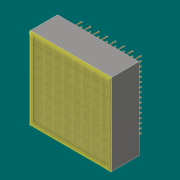
# Autodesk Inventor part: H12700A
Saved by Autodesk Inventor 2016 (Build 200138000, 138)
## iProperties
Created: 2015-10-20
Part Number: H12700A
Material: ABS Plastic
Document SubType Name: Modeling
Designer: Sawaiz
Density: 1.06 g/cm^3
Appearance: Smooth - White
Author: Sawaiz
Autodesk Inventor part; units mm, degrees
ref_plane "YZ Plane" through (0, 0, 0) normal (1, 0, 0) x (0, 1, 0)
ref_plane "XZ Plane" through (0, 0, 0) normal (0, 1, 0) x (-1, 0, 0)
ref_plane "XY Plane" through (0, 0, 0) normal (0, 0, 1) x (1, 0, 0)
sketch "Sketch1" plane through (0, 0, 0) normal (1, 0, 0) x (0, 1, 0)
  line L0 (-26, -26) -> (26, -26)
  line L1 (26, -26) -> (26, 26)
  line L2 (26, 26) -> (-26, 26)
  line L3 (-26, 26) -> (-26, -26)
  line L4 (-26, -26) -> (26, 26) construction
  line L5 (26, -26) -> (-26, 26) construction
  point P0 (0, 0)
  dimension "d0" = 52
  dimension "d1" = 52
  constraints: 12 end point, 2 midpoint, 2 parallel, 1 horizontal, 1 perpendicular
  measures "d0" distance of L2.end L1.end
  measures "d1" distance of L1.end L0.end
extrude "Extrusion1" add sketch "Sketch1" along normal blind 17.5
sketch "Sketch2" plane through (17.5, 0, 0) normal (1, 0, 0) x (0, 0, -1)
  line L0 (24.25, -24.25) -> (-24.25, -24.25)
  line L1 (-24.25, -24.25) -> (-24.25, 24.25)
  line L2 (-24.25, 24.25) -> (24.25, 24.25)
  line L3 (24.25, 24.25) -> (24.25, -24.25)
  line L4 (24.25, -24.25) -> (-24.25, 24.25) construction
  line L5 (-24.25, -24.25) -> (24.25, 24.25) construction
  point P0 (0, 0)
  dimension "d4" = 48.5
  dimension "d5" = 48.5
  constraints: 12 end point, 2 midpoint, 2 parallel, 1 horizontal, 1 perpendicular
  measures "d4" distance of L1.end L2.end
  measures "d5" distance of L0.end L1.end
extrude "Extrusion2" cut sketch "Sketch2" against normal blind 14.9
sketch "Sketch3" plane through (2.6, 0, 0) normal (1, 0, 0) x (0, 0, -1)
  line L0 (24.25, -24.25) -> (-24.25, -24.25) projected
  line L1 (24.25, 24.25) -> (24.25, -24.25) projected
  line L2 (-24.25, 24.25) -> (24.25, 24.25) projected
  line L3 (-24.25, -24.25) -> (-24.25, 24.25) projected
  line L4 (24.25, -24.25) -> (-24.25, -24.25) projected
  line L5 (-24.25, -24.25) -> (-18.1875, -24.25)
  line L6 (-18.1875, -24.25) -> (-18.1875, -18.1875)
  line L7 (-18.1875, -18.1875) -> (-24.25, -18.1875)
  line L8 (-24.25, -18.1875) -> (-24.25, -24.25)
  line L9 (-23.5764, -18.1875) -> (-22.9028, -18.1875)
  line L10 (-22.9028, -18.1875) -> (-22.9028, -24.25)
  line L11 (-22.9028, -24.25) -> (-23.5764, -24.25)
  line L12 (-23.5764, -24.25) -> (-23.5764, -18.1875)
  line L13 (-22.2292, -18.1875) -> (-21.5556, -18.1875)
  line L14 (-21.5556, -18.1875) -> (-21.5556, -24.25)
  line L15 (-21.5556, -24.25) -> (-22.2292, -24.25)
  line L16 (-22.2292, -24.25) -> (-22.2292, -18.1875)
  line L17 (-20.8819, -24.25) -> (-20.2083, -24.25)
  line L18 (-20.2083, -24.25) -> (-20.2083, -18.1875)
  line L19 (-20.2083, -18.1875) -> (-20.8819, -18.1875)
  line L20 (-20.8819, -18.1875) -> (-20.8819, -24.25)
  line L21 (-19.5347, -24.25) -> (-18.8611, -24.25)
  line L22 (-18.8611, -24.25) -> (-18.8611, -18.1875)
  line L23 (-18.8611, -18.1875) -> (-19.5347, -18.1875)
  line L24 (-19.5347, -18.1875) -> (-19.5347, -24.25)
  line L25 (-18.2875, -18.2875) -> (-18.2875, -24.15)
  line L26 (-18.2875, -24.15) -> (-24.15, -24.15)
  line L27 (-24.15, -24.15) -> (-24.15, -18.2875)
  line L28 (-24.15, -18.2875) -> (-18.2875, -18.2875)
  point P0 (0, 0)
  dimension "d8" = 6.0625
  dimension "d9" = 6.0625
  dimension "d10" = 0.6736
  dimension "d11" = 0.6736
  dimension "d12" = 0.6736
  dimension "d13" = 0.6736
  dimension "d14" = 0.6736
  dimension "d15" = 0.6736
  dimension "d16" = 0.6736
  dimension "d17" = 0.6736
  dimension "d18" = 0.1
  constraints: 48 end point, 12 parallel, 8 point on line, 6 perpendicular, 5 horizontal, 3 other
  measures "d8" distance of L7.end L6.end
  measures "d9" distance of L6.end L5.end
  measures "d10" distance between parallel lines of L8 L12
  measures "d11" distance between parallel lines of L10 L12
  measures "d12" distance between parallel lines of L10 L16
  measures "d13" distance between parallel lines of L16 L14
  measures "d14" distance between parallel lines of L14 L20
  measures "d15" distance between parallel lines of L20 L18
  measures "d16" distance between parallel lines of L18 L24
  measures "d17" distance between parallel lines of L24 L22
  measures "d18" distance between parallel lines of L6 L25
extrude "Extrusion3" add sketch "Sketch3" along normal blind 13.9 separate body contours L0 L24 L26 L22 | L26 L24 L28 L22 | L22 L28 L24 L7 | L0 L20 L26 L18 | L7 L10 L28 L12 | L26 L20 L28 L18 | L18 L28 L20 L7 | L12 L26 L10 L0 | L28 L10 L26 L12 | L0 L16 L26 L14 | L7 L14 L28 L16 | L26 L16 L28 L14
sketch "Sketch4" plane through (16.5, 0, 0) normal (1, 0, 0) x (0, 0, -1)
  line L0 (-21.5556, -24.25) -> (-21.5556, -18.1875) projected
  line L1 (-22.9028, -18.1875) -> (-23.5764, -18.1875) projected
  line L2 (-23.5764, -24.25) -> (-22.9028, -24.25) projected
  line L3 (-21.5556, -24.25) -> (-21.5556, -18.1875) projected
  line L4 (-21.5556, -18.1875) -> (-22.2292, -18.1875) projected
  line L5 (-22.2292, -24.25) -> (-21.5556, -24.25) projected
  line L6 (-20.8819, -24.25) -> (-20.2083, -24.25) projected
  line L7 (-20.2083, -18.1875) -> (-20.8819, -18.1875) projected
  line L8 (-20.8819, -18.1875) -> (-20.8819, -24.25) projected
  line L9 (-19.5347, -24.25) -> (-18.8611, -24.25) projected
  line L10 (-18.8611, -18.1875) -> (-19.5347, -18.1875) projected
  line L11 (-20.8819, -18.1875) -> (-20.8819, -24.25) projected
  line L12 (-18.1875, -24.25) -> (-24.25, -24.25)
  line L13 (-24.25, -24.25) -> (-24.25, -18.1875)
  line L14 (-24.25, -18.1875) -> (-18.1875, -18.1875)
  line L15 (-18.1875, -18.1875) -> (-18.1875, -24.25)
  line L16 (-24.15, -18.2875) -> (-24.15, -24.15)
  line L17 (-24.15, -24.15) -> (-18.2875, -24.15)
  line L18 (-18.2875, -24.15) -> (-18.2875, -18.2875)
  line L19 (-18.2875, -18.2875) -> (-24.15, -18.2875)
  line L20 (24.25, -24.25) -> (-24.25, -24.25) projected
  line L21 (-24.25, -24.25) -> (-24.25, 24.25) projected
  point P0 (0, 0)
  point P1 (-21.2188, -21.2188)
  dimension "d21" = 6.0625
  dimension "d22" = 6.0625
  dimension "d23" = 0.1
  constraints: 16 end point, 4 parallel, 2 horizontal, 2 perpendicular, 1 collinear, 4 other
  measures "d21" distance of L13.end L14.end
  measures "d22" distance of L12.end L13.end
  measures "d23" distance between parallel lines of L13 L16
extrude "Extrusion4" add sketch "Sketch4" against normal up to surface (13.9 mm away) contours L5 L12 L2 L13 L14 L1 L4 L0 L19 L16 L17 | L0 L17 L8 L12 | L8 L17 L18 L19 L7 L14 L10 L15 L12 L9 L6 | L0 L14 L8 L19 bodies 2
pattern_linear "Rectangular Pattern1" count 8 spacing 6.0625 along (0, 1, 0) count 8 spacing 6.0625 along (0, 0, -1) of "Extrusion3", "Extrusion4" bodies 2
sketch "Sketch5" plane through (17.5, 0, 0) normal (1, 0, 0) x (0, 0, -1)
  line L0 (-26, -26) -> (26, -26) projected
  line L1 (-26, 26) -> (-26, -26) projected
  line L2 (24.25, 24.25) -> (24.25, -24.25) projected
  line L3 (24.25, -24.25) -> (-24.25, -24.25) projected
  line L4 (-24.25, -24.25) -> (-24.25, 24.25) projected
  line L5 (-24.25, 24.25) -> (24.25, 24.25) projected
  line L6 (26, -26) -> (26, 26) projected
  line L7 (26, 26) -> (-26, 26) projected
  line L8 (-26, 26) -> (-26, -26) projected
  line L9 (-26, -26) -> (26, -26) projected
  point P0 (0, 0)
extrude "Extrusion5" add sketch "Sketch5" along normal blind 1.5 separate body contours L1 L7 L6 L0 | L2 L3 L4 L5
fillet "Fillet1" radius 1.5 4 edges at (19, 0, 26) (19, 26, 0) (19, 0, -26) (19, -26, 0)
sketch "Sketch7" plane through (0, 0, 0) normal (-1, 0, 0) x (0, 0, 1)
  circle A0 centre (21.3971, 18.8611) radius 0.4
  circle A1 centre (18.5441, 18.8611) radius 0.4
  line L0 (-26, -26) -> (-26, 26) projected
  line L1 (26, -26) -> (-26, -26) projected
  line L2 (26, 26) -> (26, -26) projected
  line L3 (-26, 26) -> (26, 26) projected
  line L4 (-24.25, 24.25) -> (24.25, 24.25)
  line L5 (24.25, 24.25) -> (24.25, -24.25)
  line L6 (24.25, -24.25) -> (-24.25, -24.25)
  line L7 (-24.25, -24.25) -> (-24.25, 24.25)
  line L8 (-24.25, 24.25) -> (24.25, -24.25) construction
  line L9 (24.25, 24.25) -> (-24.25, -24.25) construction
  point P0 (0, 0)
  dimension "d39" = 48.5
  dimension "d40" = 48.5
  dimension "d41" = 0.8
  dimension "d42" = 0.8
  dimension "d43" = 2.8529
  dimension "d44" = 2.8529
  dimension "d45" = 5.3889
  dimension "d46" = 5.3889
  constraints: 12 end point, 2 centre point, 2 midpoint, 2 parallel, 1 horizontal, 1 perpendicular
  measures "d39" distance of L5.end L6.end
  measures "d40" distance of L4.end L5.end
  measures "d41" diameter of A0
  measures "d42" diameter of A1
  measures "d43" distance from line of L5 A0.centre
  measures "d44" distance of A1.centre A0.centre
  measures "d45" distance from line of L4 A0.centre
  measures "d46" distance from line of L4 A1.centre
extrude "Extrusion6" add sketch "Sketch7" along normal blind 8.4 separate body contours A0 | A1
pattern_linear "Rectangular Pattern2" count 8 spacing 5.3889 along (0, -1, 0) count 8 spacing 5.7059 along (0, 0, -1) of "Extrusion6" bodies 4
equation "\"d10\" = 0.111111 * d8"
equation "\"d11\" = d10"
equation "\"d12\" = d11"
equation "\"d13\" = d12"
equation "\"d14\" = d13"
equation "\"d15\" = d14"
equation "\"d16\" = d15"
equation "\"d17\" = d16"
body "Solid1"
body "Solid2"
body "Solid3"
body "Solid4"
